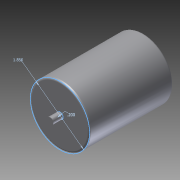
# Autodesk Inventor part: proxy 775 motor
Saved by Autodesk Inventor 2011 SP1 (Build 150282100, 282)
## iProperties
Created: 2012-01-19
Part Number: proxy 775 motor
Document SubType Name: Modeling
Designer: Christopher
Density: 1 g/cm^3
Author: Christopher
Autodesk Inventor part; units mm, degrees
ref_plane "YZ Plane" through (0, 0, 0) normal (1, 0, 0) x (0, 1, 0)
ref_plane "XZ Plane" through (0, 0, 0) normal (0, 1, 0) x (-1, 0, 0)
ref_plane "XY Plane" through (0, 0, 0) normal (0, 0, 1) x (1, 0, 0)
sketch "Sketch1" plane through (0, 0, 0) normal (0, 0, 1) x (1, 0, 0)
  circle A0 centre (0, 0) radius 23.495
  circle A1 centre (0, 0) radius 2.54
  dimension "d0" = 46.99
  dimension "d3" = 5.08
  constraints: 3 coincident, 2 centre point
  measures "d0" diameter of A0
  measures "d3" diameter of A1
extrude "Extrusion1" add sketch "Sketch1" against normal blind 66.548 contours A0 | A1
extrude "Extrusion2" add sketch "Sketch1" along normal blind 7.62 contours A1
fillet "Fillet1" radius 1.5875 1 edges at (-23.495, 0, 0)
fillet "Fillet2" radius 1.5875 1 edges at (-23.495, 0, -66.548)
body "Solid1"
